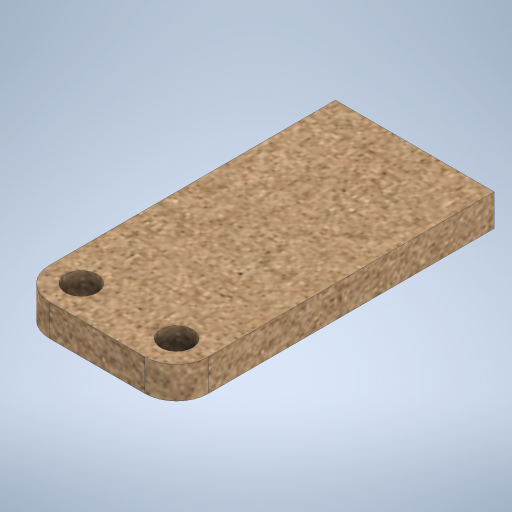
# Autodesk Inventor part: DedoV2
Saved by Autodesk Inventor 2023.1 (Build 271208000, 208)
## iProperties
Created: 2022-10-30
Part Number: DedoV2
Material: MDF Medium Density Fiberboard
Document SubType Name: Modeling
Designer: Daniel Peña
Density: 0.8 g/cm^3
Appearance: Cardboard - Corrugated
Author: Daniel Peña
Autodesk Inventor part; units mm, degrees
ref_plane "YZ Plane" through (0, 0, 0) normal (1, 0, 0) x (0, 1, 0)
ref_plane "XZ Plane" through (0, 0, 0) normal (0, 1, 0) x (-1, 0, 0)
ref_plane "XY Plane" through (0, 0, 0) normal (0, 0, 1) x (1, 0, 0)
sketch "Sketch1" plane through (0, 0, 0) normal (0, 0, 1) x (1, 0, 0)
  line L0 (-20, 12.5) -> (25, 12.5)
  line L1 (25, 12.5) -> (25, -12.5)
  line L2 (25, -12.5) -> (-20, -12.5)
  line L3 (-25, -7.5) -> (-25, 7.5)
  arc A0 (-20, 12.5) -> (-25, 7.5) centre (-20, 7.5) ccw
  arc A1 (-25, -7.5) -> (-20, -12.5) centre (-20, -7.5) ccw
  point P0 (0, 0)
  point P1 (-25, 12.5)
  point P2 (-25, -12.5)
  dimension "d0" = 25
  dimension "d1" = 50
  dimension "d2" = 5
  dimension "d5" = 12.5
  dimension "d6" = 25
  constraints: 8 end point, 4 point on circle, 4 point on line, 4 tangent, 2 centre point, 2 parallel, 1 equal radius, 1 horizontal, 1 perpendicular
  measures "d0" distance of point (-25, -12.5) point (-25, 12.5)
  measures "d1" distance of point (-25, 12.5) L0.end
  measures "d2" radius of A0
  measures "d5" distance from line of point (0, 0) L0
  measures "d6" distance from line of L3 point (0, 0)
extrude "Extrusion1" add sketch "Sketch1" along normal blind 5
sketch "Sketch2" plane through (0, 0, 5) normal (0, 0, 1) x (1, 0, 0)
  arc A0 (-20, 12.5) -> (-25, 7.5) centre (-20, 7.5) ccw projected
  arc A1 (-25, -7.5) -> (-20, -12.5) centre (-20, -7.5) ccw projected
  point P0 (0, 0)
  constraints: 2 coincident
hole "Hole1" at (-20, 7.5, 5) at (-20, -7.5, 5) direction (0, 0, -1) diameter 5 end through all
body "Solid1"
